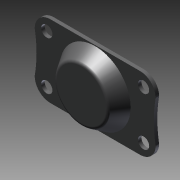
# Autodesk Inventor part: CHAMJ-E50-Rswivel
Saved by Autodesk Inventor 2015 (Build 190159000, 159)
## iProperties
Category: PARTsolutions
Company: MISUMI
Created: 2015-12-24
Part Number: CHAMJ-E50-Rswivel
Catalog Web Link: www.cadenas.de
Description: CHAMJ_E, CHAMK_E, CHAMS_Eswivel-Caster
Vendor: MISUMI
Document SubType Name: Modeling
Designer: psAdmin
Manufacturer: MISUMI
Mass: 12.6071 g
Surface Area: 65.6489 cm^2
Volume: 12.6071 cm^3
Density: 1 g/cm^3
Material: 一般
Appearance: PSOLRGB-192-192-192
PSOL_IDENT_0: {$CADENAS_DATA\23d-libs\misumi\metric\42_casters_leveling_pads\chamj_e_swivel.prj},210 {VTYP=3D},{NB=
PSOL_IDENT_1: CHAMJ-E50-Rswivel},{LINA=CHAMJ-E50-Rswivel},{NN=CHAMJ_E, CHAMK_E, CHAMS_Eswivel},{DATE=05.06.2015 05
PSOL_IDENT_2: :25:13},{GEOMDATE=03.09.2009 00:00:00},{VERSION=},{LINEID=30},{LINESUBID=-1},{WBVAR=TSMB,MATW}  {NB=
PSOL_IDENT_3: CHAMJ-E50-Rswivel},{LINA=CHAMJ-E50-Rswivel},{KT=DUMMY},{PN=CHAMJ-E50-R},{TYPE=CHAMJ-E},{TSMB=1},{MAT
PSOL_IDENT_4: MB=Low Carbon Steel},{STMB=Trivalnt Chromate},{D=50},{MATW=R},{COLORW=Black},{BSP=Available},{BWP=No
PSOL_IDENT_5: t Available},{H=65},{A=70},{C=42},{F1=56},{F2=28},{DD=6.5},{E=22},{RR=47},{B=20},{TT=2.0},{BR=20},{B
PSOL_IDENT_6: U=21},{BN=21},{AL=300},{ALR=300},{ALU=380},{ALN=400},{MASS=180}
NN: CHAMJ_E, CHAMK_E, CHAMS_Eswivel
NT: Caster
NB: CHAMJ-E50-Rswivel
NBSYN: $PN.swivel
LINA: CHAMJ-E50-Rswivel
PN: CHAMJ-E50-R
TSMB: Swivel
MATMB: Low Carbon Steel
STMB: Trivalnt Chromate
D: 50
MATW: Synthetic Rubber
COLORW: Black
BSP: Available
BWP: Not Available
H: 65
A: 70
C: 42
F1: 56
F2: 28
DD: 6.5
E: 22
RR: 47
B: 20
TT: 2.0
AL: 300
MASS: 180
SUPPLIER: MISUMI
ARTICLENO: CHAMJ-E50-Rswivel
BOMINFO: CHAMJ-E50-Rswivel
CREATOR: CADENAS GmbH
Title: CHAMJ-E50-Rswivel
Author: Cadenas PARTsolutions
Comments: Caster
Autodesk Inventor part; units mm, degrees
sketch "Sketch_1" plane through (0, 0, 0) normal (0, 1, 0) x (-1, 0, 0)
  arc A0 (35, 12) -> (35, -12) centre (103.9638, 0) ccw
  arc A1 (35, 12) -> (26, 21) centre (26, 12) ccw
  line L0 (26, 21) -> (-26, 21)
  arc A2 (-26, 21) -> (-35, 12) centre (-26, 12) ccw
  arc A3 (-35, -12) -> (-35, 12) centre (-103.9638, 0) ccw
  arc A4 (-35, -12) -> (-26, -21) centre (-26, -12) ccw
  line L1 (-26, -21) -> (26, -21)
  arc A5 (26, -21) -> (35, -12) centre (26, -12) ccw
  circle A6 centre (-28, 14) radius 3.25
  circle A7 centre (-28, -14) radius 3.25
  circle A8 centre (28, 14) radius 3.25
  circle A9 centre (28, -14) radius 3.25
  constraints: 12 point on circle, 10 centre point, 4 end point
extrude "Extrusion1" add sketch "Sketch_1" against normal blind 2
sketch "Sketch2" plane through (0, 0, 0) normal (0, 1, 0) x (1, 0, 0)
  point P0 (0, 0)
hole "Hole1" at (0, 0, 0) direction (0, -1, 0) diameter 33.6 depth 1
sketch "Sketch_4" plane through (0, 0, 0) normal (0, 0, 1) x (1, 0, 0)
  line L0 (0, -10) -> (0, -2)
  line L1 (0, -2) -> (20.5, -2)
  line L2 (20.5, -2) -> (15.8744, -9.0925)
  arc A0 (14.1992, -10) -> (15.8744, -9.0925) centre (14.1992, -8) ccw
  line L3 (14.1992, -10) -> (0, -10)
  line L4 (0, -10) -> (0, -2)
  constraints: 10 end point, 2 point on circle, 1 centre point
revolve "Revolution1" add sketch "Sketch_4" angle 360 about axis through (0, -10, 0) along (0, -1, 0)
ref_plane "swivel_to_body_XY" through (0, -10, 0) normal (0, 1, 0) x (1, 0, 0)
ref_plane "swivel_to_body_YZ" through (0, -10, 0) normal (1, 0, 0) x (0, 0, -1)
ref_plane "swivel_to_body_ZX" through (0, -10, 0) normal (0, 0, -1) x (0, 1, 0)
body "Solid1"
